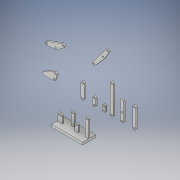
# Autodesk Inventor part: 二連趕
Saved by Autodesk Inventor 2017 (Build 210142000, 142)
## iProperties
Part Number: 二連趕
Material: 一般
Document SubType Name: Modeling
Designer: 士正
Density: 1 g/cm^3
Appearance: 預設
Author: 士正
Autodesk Inventor part; units mm, degrees
ref_plane "YZ Plane" through (0, 0, 0) normal (1, 0, 0) x (0, 1, 0)
ref_plane "XZ Plane" through (0, 0, 0) normal (0, 1, 0) x (-1, 0, 0)
sketch "草圖1" plane through (0, 0, 0) normal (0, 1, 0) x (-1, 0, 0)
  line L0 (-35.5444, 25.4936) -> (-35.5444, 0)
  line L1 (-57.9223, 11.8756) -> (-57.9223, 0)
  line L2 (-77.0101, 7.1505) -> (-77.0101, 0)
  line L3 (-92.1051, 53.0302) -> (-92.1051, 0)
  line L4 (-112.1667, 34.3593) -> (-112.1667, 0)
  line L5 (-136.1239, 35.4232) -> (-136.1239, 0)
  line L6 (-35.5444, 0) -> (-35.5444, 25.4936) construction
  line L7 (-32.5444, 0) -> (-32.5444, 25.4936)
  line L8 (-38.5444, 25.4936) -> (-38.5444, 0)
  arc A0 (-38.5444, 0) -> (-32.5444, 0) centre (-35.5444, 0) ccw
  arc A1 (-32.5444, 25.4936) -> (-38.5444, 25.4936) centre (-35.5444, 25.4936) ccw
  line L9 (-57.9223, 11.8756) -> (-57.9223, 0) construction
  line L10 (-60.9223, 11.8756) -> (-60.9223, 0)
  line L11 (-54.9223, 0) -> (-54.9223, 11.8756)
  arc A2 (-54.9223, 11.8756) -> (-60.9223, 11.8756) centre (-57.9223, 11.8756) ccw
  arc A3 (-60.9223, 0) -> (-54.9223, 0) centre (-57.9223, 0) ccw
  line L12 (-77.0101, 7.1505) -> (-77.0101, 0) construction
  line L13 (-80.0101, 7.1505) -> (-80.0101, 0)
  line L14 (-74.0101, 0) -> (-74.0101, 7.1505)
  arc A4 (-74.0101, 7.1505) -> (-80.0101, 7.1505) centre (-77.0101, 7.1505) ccw
  arc A5 (-80.0101, 0) -> (-74.0101, 0) centre (-77.0101, 0) ccw
  line L15 (-92.1051, 0) -> (-92.1051, 53.0302) construction
  line L16 (-89.1051, 0) -> (-89.1051, 53.0302)
  line L17 (-95.1051, 53.0302) -> (-95.1051, 0)
  arc A6 (-95.1051, 0) -> (-89.1051, 0) centre (-92.1051, 0) ccw
  arc A7 (-89.1051, 53.0302) -> (-95.1051, 53.0302) centre (-92.1051, 53.0302) ccw
  line L18 (-112.1667, 34.3593) -> (-112.1667, 0) construction
  line L19 (-115.1667, 34.3593) -> (-115.1667, 0)
  line L20 (-109.1667, 0) -> (-109.1667, 34.3593)
  arc A8 (-109.1667, 34.3593) -> (-115.1667, 34.3593) centre (-112.1667, 34.3593) ccw
  arc A9 (-115.1667, 0) -> (-109.1667, 0) centre (-112.1667, 0) ccw
  line L21 (-136.1239, 0) -> (-136.1239, 35.4232) construction
  line L22 (-133.1239, 0) -> (-133.1239, 35.4232)
  line L23 (-139.1239, 35.4232) -> (-139.1239, 0)
  arc A10 (-139.1239, 0) -> (-133.1239, 0) centre (-136.1239, 0) ccw
  arc A11 (-133.1239, 35.4232) -> (-139.1239, 35.4232) centre (-136.1239, 35.4232) ccw
  point P0 (0, 0)
  point P1 (-35.5444, 12.7468)
  point P2 (-57.9223, 5.9378)
  point P3 (-77.0101, 3.5753)
  point P4 (-92.1051, 26.5151)
  point P5 (-112.1667, 17.1797)
  point P6 (-136.1239, 17.7116)
  dimension "d0" = 35.4232
  dimension "d1" = 34.3593
  dimension "d2" = 53.0302
  dimension "d3" = 7.1505
  dimension "d4" = 11.8756
  dimension "d5" = 25.4936
  dimension "d6" = 3
  dimension "d7" = 35.5444
  dimension "d8" = 22.3778
  dimension "d9" = 41.4656
  dimension "d10" = 56.5606
  dimension "d11" = 76.6223
  dimension "d12" = 100.5795
  constraints: 60 end point, 24 point on circle, 24 tangent, 12 centre point, 12 equal length, 6 horizontal alignment, 6 midpoint, 6 vertical, 5 equal radius
  measures "d0" distance of L5.start L5.end
  measures "d1" distance of L4.start L4.end
  measures "d2" distance of L3.start L3.end
  measures "d3" distance of L2.start L2.end
  measures "d4" distance of L1.start L1.end
  measures "d5" distance of L0.start L0.end
  measures "d6" radius of A1
  measures "d7" distance from line of point (0, 0) L0
  measures "d8" distance between parallel lines of L0 L9
  measures "d9" distance between parallel lines of L0 L12
  measures "d10" distance between parallel lines of L0 L15
  measures "d11" distance between parallel lines of L0 L18
  measures "d12" distance between parallel lines of L0 L21
extrude "擠出1" add sketch "草圖1" along normal mid plane 3 contours A4 L14 A5 L13
extrude "擠出5" add sketch "草圖1" along normal mid plane 3 separate body contours A0 L8 A1 L7
extrude "擠出6" add sketch "草圖1" along normal mid plane 3 separate body contours A2 L11 A3 L10
extrude "擠出7" add sketch "草圖1" along normal mid plane 3 separate body contours A6 L17 A7 L16
extrude "擠出8" add sketch "草圖1" along normal mid plane 3 separate body contours A8 L20 A9 L19
extrude "擠出9" add sketch "草圖1" along normal mid plane 3 separate body contours A10 L23 A11 L22
sketch "草圖2" plane through (0, 0, 0) normal (0, 1, 0) x (-1, 0, 0)
  line L0 (34.405, 6.7684) -> (17.2512, 14.6099)
  line L1 (17.2512, 14.6099) -> (20.1637, 4.8695)
  line L2 (20.1637, 4.8695) -> (34.405, 6.7684)
  line L3 (18.4984, 17.3384) -> (40.1997, 7.418)
  line L4 (38.9237, 1.6897) -> (20.135, 1.8696)
  line L5 (17.2894, 4.01) -> (14.3769, 13.7505)
  arc A0 (17.2894, 4.01) -> (20.135, 1.8696) centre (20.1637, 4.8695) ccw
  arc A1 (18.4984, 17.3384) -> (14.3769, 13.7505) centre (17.2512, 14.6099) ccw
  arc A2 (38.9237, 1.6897) -> (40.1997, 7.418) centre (38.9524, 4.6896) ccw
  line L6 (33.7973, 58.2107) -> (2.9521, 69.37)
  line L7 (2.9521, 69.37) -> (16.7345, 59.1184)
  line L8 (16.7345, 59.1184) -> (33.7973, 58.2107)
  line L9 (-75.3929, 89.8027) -> (-84.0644, 104.2867)
  line L10 (-84.0644, 104.2867) -> (-58.0761, 69.9708)
  line L11 (-58.0761, 69.9708) -> (-75.3929, 89.8027)
  line L12 (-55.6846, 71.782) -> (-81.6728, 106.0979)
  line L13 (-86.6384, 102.7457) -> (-77.9669, 88.2617)
  line L14 (-77.6527, 87.8295) -> (-60.3359, 67.9976)
  arc A3 (-60.3359, 67.9976) -> (-55.6846, 71.782) centre (-58.0761, 69.9708) ccw
  arc A4 (-81.6728, 106.0979) -> (-86.6384, 102.7457) centre (-84.0644, 104.2867) ccw
  arc A5 (-77.9669, 88.2617) -> (-77.6527, 87.8295) centre (-75.3929, 89.8027) ccw
  line L15 (3.9727, 72.1911) -> (34.8179, 61.0318)
  line L16 (33.638, 55.215) -> (16.5752, 56.1226)
  line L17 (14.9441, 56.7113) -> (1.1617, 66.9629)
  arc A6 (33.638, 55.215) -> (34.8179, 61.0318) centre (33.7973, 58.2107) ccw
  arc A7 (14.9441, 56.7113) -> (16.5752, 56.1226) centre (16.7345, 59.1184) ccw
  arc A8 (3.9727, 72.1911) -> (1.1617, 66.9629) centre (2.9521, 69.37) ccw
  point P0 (0, 0)
  point P1 (-77.8291, 88.0316)
  dimension "d15" = 18.8612
  dimension "d17" = 10.1666
  dimension "d18" = 14.3674
  dimension "d19" = 3
  dimension "d20" = 3
  dimension "d21" = 3
  dimension "d23" = 17.0869
  dimension "d24" = 17.177
  dimension "d25" = 32.8017
  dimension "d28" = 26.3282
  dimension "d29" = 16.8814
  dimension "d30" = 43.0462
  dimension "d31" = 3
  dimension "d32" = 3
  dimension "d50" = 3
  dimension "d101" = 3
  dimension "d102" = 3
  dimension "d104" = 5
  constraints: 36 end point, 18 point on circle, 18 tangent, 9 centre point, 5 point on line, 4 equal radius, 4 other
  measures "d15" distance of L0.start L0.end
  measures "d17" distance of L0.end L1.end
  measures "d18" distance of L1.end L0.start
  measures "d19" distance between parallel lines of L1 L5
  measures "d20" radius of A0
  measures "d21" radius of A2
  measures "d23" distance of L7.end L6.start
  measures "d24" distance of L6.end L7.end
  measures "d25" distance of L6.start L6.end
  measures "d28" distance of L10.end L9.start
  measures "d29" distance of L9.start L9.end
  measures "d30" distance of L9.end L10.end
  measures "d31" distance between parallel lines of L9 L13
  measures "d32" radius of A3
  measures "d50" radius of A5
  measures "d101" distance between parallel lines of L15 L6
  measures "d102" radius of A6
  measures "d104" distance of A2.centre L0.start
extrude "擠出2" add sketch "草圖2" along normal mid plane 3 separate body contours L2 L1 L0 | L3 A2 L4 A0 L5 A1
extrude "擠出10" add sketch "草圖2" along normal mid plane 3 separate body contours L8 L7 L6 | L15 A6 L16 A7 L17 A8
extrude "擠出11" add sketch "草圖2" along normal mid plane 3 separate body contours L9 L10 L11 | A3 L14 A5 L13 A4 L12
sketch "草圖3" plane through (0, 0, 0) normal (0, 1, 0) x (-1, 0, 0)
  arc A0 (8.4634, -52.7511) -> (8.4634, -48.0489) centre (10.3269, -50.4) ccw
  arc A1 (8.4634, -48.0489) -> (8.4634, -52.7511) centre (6.6, -50.4) ccw
  circle A2 centre (-10.2, -40) radius 3
  circle A3 centre (-23.8, -50.4) radius 3
  circle A4 centre (-43.78, -30.23) radius 3
  line L0 (13.3269, -50.4) -> (13.3269, -62.4)
  line L1 (3.6, -50.4) -> (3.6, -62.4)
  line L2 (-7.2, -40) -> (-7.2, -62.4)
  line L3 (-13.2, -40) -> (-13.2, -62.4)
  line L4 (-20.8, -50.4) -> (-20.8, -62.4)
  line L5 (-26.8, -50.4) -> (-26.8, -62.4)
  line L6 (-40.78, -30.23) -> (-40.78, -62.4)
  line L7 (-46.78, -30.23) -> (-46.78, -62.4)
  line L8 (13.3269, -62.4) -> (-46.78, -62.4)
  line L9 (-46.78, -62.4) -> (-46.78, -67.4)
  line L10 (-46.78, -67.4) -> (13.3269, -67.4)
  line L11 (13.3269, -67.4) -> (13.3269, -62.4)
  point P0 (0, 0)
  dimension "d35" = 6
  dimension "d36" = 6.6
  dimension "d37" = 10.3269
  dimension "d38" = 10.4
  dimension "d39" = 10.2
  dimension "d40" = 23.8
  dimension "d41" = 20.17
  dimension "d42" = 43.78
  dimension "d43" = 40
  dimension "d44" = 12
  dimension "d45" = 5
  constraints: 24 end point, 12 point on circle, 7 tangent, 7 vertical, 6 point on line, 5 centre point, 4 equal radius, 2 horizontal alignment, 2 parallel, 1 horizontal, 1 perpendicular
  measures "d35" diameter of A1
  measures "d36" horizontal distance of point (0, 0) A1.centre
  measures "d37" horizontal distance of point (0, 0) A0.centre
  measures "d38" vertical distance of A0.centre A2.centre
  measures "d39" horizontal distance of point (0, 0) A2.centre
  measures "d40" horizontal distance of point (0, 0) A3.centre
  measures "d41" vertical distance of A3.centre A4.centre
  measures "d42" horizontal distance of point (0, 0) A4.centre
  measures "d43" vertical distance of point (0, 0) A2.centre
  measures "d44" distance of L0.start L0.end
  measures "d45" distance of L10.end L0.end
extrude "擠出3" add sketch "草圖3" along normal mid plane 3 separate body contours A1 A0 | A0 L0 L8 L1 A1 | L7 A4 L6 L8 | L8 L5 A3 L4 | A4 | A3
extrude "擠出12" add sketch "草圖3" along normal mid plane 25 separate body contours L11 L10 L9 L8
ref_plane "工作平面1" through (0, 4.5, 0) normal (0, -1, 0) x (1, 0, 0)
sketch "草圖7" plane through (0, 4.5, 0) normal (0, -1, 0) x (1, 0, 0)
  line L0 (7.2, -40) -> (7.2, -62.4) projected
  line L1 (13.2, -40) -> (13.2, -62.4) projected
  circle A0 centre (10.2, -40) radius 3 projected
  line L2 (7.2, -62.4) -> (13.2, -62.4)
  line L3 (-13.3269, -62.4) -> (46.78, -62.4) projected
  point P0 (0, 0)
  constraints: 2 end point, 1 collinear
extrude "擠出13" add sketch "草圖7" against normal blind 3 separate body
combine bodies "合併1" operation type add bodies to combine 11 10
combine bodies "合併2" operation type add bodies to combine 12 11
sketch "草圖6" plane through (0, -1.5, 0) normal (0, -1, 0) x (1, 0, 0)
  arc A0 (80.0101, 7.1505) -> (74.0101, 7.1505) centre (77.0101, 7.1505) ccw projected
  line L0 (80.0101, 7.1505) -> (80.0101, 0) projected
  arc A1 (74.0101, 0) -> (80.0101, 0) centre (77.0101, 0) ccw projected
  line L1 (74.0101, 0) -> (74.0101, 7.1505) projected
  arc A2 (32.5444, 0) -> (38.5444, 0) centre (35.5444, 0) ccw projected
  line L2 (32.5444, 0) -> (32.5444, 25.4936) projected
  arc A3 (38.5444, 25.4936) -> (32.5444, 25.4936) centre (35.5444, 25.4936) ccw projected
  line L3 (38.5444, 25.4936) -> (38.5444, 0) projected
  arc A4 (60.9223, 11.8756) -> (54.9223, 11.8756) centre (57.9223, 11.8756) ccw projected
  line L4 (60.9223, 11.8756) -> (60.9223, 0) projected
  arc A5 (54.9223, 0) -> (60.9223, 0) centre (57.9223, 0) ccw projected
  line L5 (54.9223, 0) -> (54.9223, 11.8756) projected
  arc A6 (89.1051, 0) -> (95.1051, 0) centre (92.1051, 0) ccw projected
  line L6 (89.1051, 0) -> (89.1051, 53.0302) projected
  arc A7 (95.1051, 53.0302) -> (89.1051, 53.0302) centre (92.1051, 53.0302) ccw projected
  line L7 (95.1051, 53.0302) -> (95.1051, 0) projected
  arc A8 (115.1667, 34.3593) -> (109.1667, 34.3593) centre (112.1667, 34.3593) ccw projected
  line L8 (115.1667, 34.3593) -> (115.1667, 0) projected
  arc A9 (109.1667, 0) -> (115.1667, 0) centre (112.1667, 0) ccw projected
  line L9 (109.1667, 0) -> (109.1667, 34.3593) projected
  arc A10 (133.1239, 0) -> (139.1239, 0) centre (136.1239, 0) ccw projected
  line L10 (133.1239, 0) -> (133.1239, 35.4232) projected
  arc A11 (139.1239, 35.4232) -> (133.1239, 35.4232) centre (136.1239, 35.4232) ccw projected
  line L11 (139.1239, 35.4232) -> (139.1239, 0) projected
  arc A12 (-14.3769, 13.7505) -> (-18.4984, 17.3384) centre (-17.2512, 14.6099) ccw projected
  line L12 (-14.3769, 13.7505) -> (-17.2894, 4.01) projected
  arc A13 (-20.135, 1.8696) -> (-17.2894, 4.01) centre (-20.1637, 4.8695) ccw projected
  line L13 (-20.135, 1.8696) -> (-38.9237, 1.6897) projected
  arc A14 (-40.1997, 7.418) -> (-38.9237, 1.6897) centre (-38.9524, 4.6896) ccw projected
  line L14 (-40.1997, 7.418) -> (-18.4984, 17.3384) projected
  arc A15 (55.6846, 71.782) -> (60.3359, 67.9976) centre (58.0761, 69.9708) ccw projected
  line L15 (55.6846, 71.782) -> (81.6728, 106.0979) projected
  arc A16 (86.6384, 102.7457) -> (81.6728, 106.0979) centre (84.0644, 104.2867) ccw projected
  line L16 (86.6384, 102.7457) -> (77.9669, 88.2617) projected
  arc A17 (77.6527, 87.8295) -> (77.9669, 88.2617) centre (75.3929, 89.8027) ccw projected
  line L17 (77.6527, 87.8295) -> (60.3359, 67.9976) projected
  line L18 (-3.6, -62.4) -> (20.8, -62.4) projected
  line L19 (-13.3269, -62.4) -> (-3.6, -62.4) projected
  line L20 (-13.3269, -67.4) -> (-13.3269, -62.4) projected
  line L21 (46.78, -67.4) -> (-13.3269, -67.4) projected
  line L22 (46.78, -62.4) -> (46.78, -67.4) projected
  line L23 (26.8, -62.4) -> (40.78, -62.4) projected
  line L24 (-3.6, -50.4) -> (-3.6, -62.4) projected
  arc A18 (-3.6, -50.4) -> (-8.4634, -48.0489) centre (-6.6, -50.4) ccw projected
  arc A19 (-8.4634, -48.0489) -> (-13.3269, -50.4) centre (-10.3269, -50.4) ccw projected
  line L25 (-13.3269, -62.4) -> (-13.3269, -50.4) projected
  line L26 (46.78, -30.23) -> (46.78, -62.4) projected
  arc A20 (46.78, -30.23) -> (40.78, -30.23) centre (43.78, -30.23) ccw projected
  line L27 (40.78, -62.4) -> (40.78, -30.23) projected
  line L28 (26.8, -50.4) -> (26.8, -62.4) projected
  arc A21 (26.8, -50.4) -> (20.8, -50.4) centre (23.8, -50.4) ccw projected
  line L29 (20.8, -62.4) -> (20.8, -50.4) projected
  line L30 (40.78, -62.4) -> (46.78, -62.4) projected
  line L31 (20.8, -62.4) -> (26.8, -62.4) projected
  arc A22 (-16.5752, 56.1226) -> (-14.9441, 56.7113) centre (-16.7345, 59.1184) ccw projected
  line L32 (-16.5752, 56.1226) -> (-33.638, 55.215) projected
  arc A23 (-34.8179, 61.0318) -> (-33.638, 55.215) centre (-33.7973, 58.2107) ccw projected
  line L33 (-34.8179, 61.0318) -> (-3.9727, 72.1911) projected
  arc A24 (-1.1617, 66.9629) -> (-3.9727, 72.1911) centre (-2.9521, 69.37) ccw projected
  line L34 (-1.1617, 66.9629) -> (-14.9441, 56.7113) projected
  point P0 (0, 0)
  point P1 (-16.9136, 59.0768)
  point P2 (10.2, -40)
  point P3 (-16.9136, 59.0768)
  point P4 (10.2, -40)
  point P5 (112.1667, 15.0398)
  dimension "d95" = 15.0398
  constraints: 24 coincident, 1 vertical alignment
  measures "d95" distance of point (112.167, 0) point (112.167, 15.04)
hole "孔4" at (-16.9136, -1.5, 59.0768) at (58.0761, -1.5, 69.9708) at (84.0644, -1.5, 104.2867) at (75.3929, -1.5, 89.8027) at (136.1239, -1.5, 35.4232) at (136.1239, -1.5, 0) at (112.1667, -1.5, 0) at (92.1051, -1.5, 53.0302) at (92.1051, -1.5, 0) at (77.0101, -1.5, 0) at (77.0101, -1.5, 7.1505) at (57.9223, -1.5, 0) at (57.9223, -1.5, 11.8756) at (35.5444, -1.5, 25.4936) at (35.5444, -1.5, 0) at (-20.1637, -1.5, 4.8695) at (-17.2512, -1.5, 14.6099) at (-10.3269, -1.5, -50.4) at (-6.6, -1.5, -50.4) at (10.2, -1.5, -40) at (23.8, -1.5, -50.4) at (43.78, -1.5, -30.23) at (112.1667, -1.5, 15.0398) at (-2.9521, -1.5, 69.37) at (-33.7973, -1.5, 58.2107) direction (0, 1, 0) diameter 3 end through all bodies 7 2 12 3 1 4 5 6 9 8
